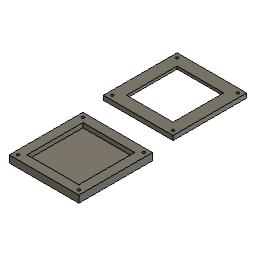
SabhyaPad Case Cut (Autodesk Fusion 360 design; units mm, degrees)
part number: 2026-05-18-20-34-42-507
Autodesk Fusion 360 part; units mm, degrees
sketch "Sketch2" plane through (0, 0, 0) normal (0, 1, 0) x (1, 0, 0)
  line L0 (-39.0756, 20.5112) -> (18.6744, 20.5112)
  line L1 (18.6744, 20.5112) -> (18.6744, -41.7388)
  line L2 (18.6744, -41.7388) -> (-39.0756, -41.7388)
  line L3 (-39.0756, -41.7388) -> (-39.0756, 20.5112)
  line L4 (-49.0756, 30.5112) -> (28.6744, 30.5112)
  line L5 (28.6744, 30.5112) -> (28.6744, -51.7388)
  line L6 (28.6744, -51.7388) -> (-49.0756, -51.7388)
  line L7 (-49.0756, -51.7388) -> (-49.0756, 30.5112)
  circle A0 centre (-44.0756, 25.5112) radius 1.45
  circle A1 centre (-44.0756, -46.7388) radius 1.45
  circle A2 centre (23.6744, -46.7388) radius 1.45
  circle A3 centre (23.6744, 25.5112) radius 1.45
  line L8 (-36.0756, 17.5112) -> (15.6744, 17.5112)
  line L9 (15.6744, 17.5112) -> (15.6744, -38.7388)
  line L10 (15.6744, -38.7388) -> (-36.0756, -38.7388)
  line L11 (-36.0756, -38.7388) -> (-36.0756, 17.5112)
  dimension "d31" = 57.75
  dimension "d32" = 62.25
  dimension "d35" = 10
  dimension "d36" = 10
  dimension "d37" = 10
  dimension "d38" = 10
  dimension "d39" = 2.9
  dimension "d40" = 5
  dimension "d41" = 5
  dimension "d42" = 2.9
  dimension "d43" = 5
  dimension "d45" = 5
  dimension "d46" = 2.9
  dimension "d47" = 5
  dimension "d48" = 5
  dimension "d49" = 2.9
  dimension "d50" = 5
  dimension "d51" = 5
  dimension "d83" = 51.75
  dimension "d84" = 56.25
  dimension "d85" = 3
  dimension "d86" = 3
  dimension "d87" = 3
  dimension "d88" = 3
  constraint horizontal L0
  constraint vertical L1
  constraint horizontal L2
  constraint vertical L3
  constraint horizontal L4
  constraint vertical L5
  constraint horizontal L6
  constraint vertical L7
  constraint horizontal L8
  constraint vertical L9
  constraint horizontal L10
  constraint vertical L11
  measures "d31" distance of L0.start L0.end
  measures "d32" distance of L0.start L2.end
  measures "d35" distance of L0 L4
  measures "d36" distance of L2 L6
  measures "d37" distance of L1 L5
  measures "d38" distance of L3 L7
  measures "d39" diameter of A0
  measures "d40" distance of L4 A0.centre
  measures "d41" distance of L7 A0.centre
  measures "d42" diameter of A1
  measures "d43" distance of L7 A1.centre
  measures "d45" distance of L6 A1.centre
  measures "d46" diameter of A2
  measures "d47" distance of L5 A2.centre
  measures "d48" distance of L6 A2.centre
  measures "d49" diameter of A3
  measures "d50" distance of L5 A3.centre
  measures "d51" distance of L4 A3.centre
  measures "d83" distance of L8.start L8.end
  measures "d84" distance of L8.start L10.end
  measures "d85" distance of L3 L11
  measures "d86" distance of L0 L8
  measures "d87" distance of L1 L9
  measures "d88" distance of L2 L10
extrude "Extrude14" add sketch "Sketch2" along normal blind 13 contours L0 L1 L2 L3 makes body 1
move_body "Move12" bodies 1 to x (1, 0, 0) y (0, 1, 0) z (0, 0, 1) at (0, -3, 0)
extrude "Extrude15" cut sketch "Sketch2" along normal blind 7 contours L0 L1 L2 L3 bodies 1 makes body 2 at (-38.0756, -3, 19.9888)
extrude "Extrude16" add sketch "Sketch2" against normal blind 3 contours L8 L9 L10 L11 bodies 2
move_body "Move13" bodies 1 2 to x (1, 0, 0) y (0, 1, 0) z (0, 0, 1) at (0, 3, 0)
extrude "Extrude17" add sketch "Sketch2" along normal blind 13 contours L4 L5 L6 L7 bodies 1 2
split "Split1" by plane through (-10.2006, 8, 10.6138) normal (0, 1, 0) bodies 1 makes body 3 at (-41.9344, 13, 1.2388)
move_body "Move14" bodies 1 to x (1, 0, 0) y (0, 1, 0) z (0, 0, 1) at (0, 0, 105)
